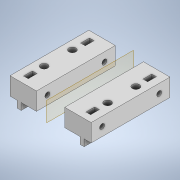
# Autodesk Inventor part: kątnik_v2
Saved by Autodesk Inventor 2022.3 (Build 263350000, 350)
## iProperties
Created: 2022-07-31
Part Number: kątnik_v2
Material: Generic
Document SubType Name: Modeling
Designer: komputer
Density: 1 g/cm^3
Appearance: Default
Author: komputer
Autodesk Inventor part; units mm, degrees
ref_plane "YZ Plane" through (0, 0, 0) normal (1, 0, 0) x (0, 1, 0)
ref_plane "XZ Plane" through (0, 0, 0) normal (0, 1, 0) x (-1, 0, 0)
ref_plane "XY Plane" through (0, 0, 0) normal (0, 0, 1) x (1, 0, 0)
sketch "Sketch1" plane through (0, 0, 0) normal (0, 0, 1) x (1, 0, 0)
  line L0 (1.5, 3.5) -> (1.5, -11.5)
  line L1 (14.5, -11.5) -> (1.5, -11.5)
  line L2 (14.5, -17.3) -> (14.5, -11.5)
  line L3 (18, -17.3) -> (14.5, -17.3)
  line L4 (18, -11.5) -> (18, -17.3)
  line L5 (24, -11.5) -> (18, -11.5)
  line L6 (24, 3.5) -> (24, -11.5)
  line L7 (1.5, 3.5) -> (24, 3.5)
  point P0 (0, 0)
  point P1 (0, 0)
  constraints: 16 end point
extrude "Extrusion1" add sketch "Sketch1" along normal blind 100
sketch "Sketch2" plane through (1.5, -11.5, 0) normal (0, -1, 0) x (1, 0, 0)
  line L0 (0, 0) -> (13, 0) projected
  line L1 (13, 0) -> (13, 100) projected
  line L2 (0, 100) -> (13, 100) projected
  line L3 (0, 0) -> (0, 100) projected
  line L4 (16.5, 0) -> (22.5, 0) projected
  line L5 (22.5, 0) -> (22.5, 100) projected
  line L6 (16.5, 100) -> (22.5, 100) projected
  line L7 (16.5, 0) -> (16.5, 100) projected
  line L8 (22.5, 61) -> (22.5, 0)
  line L9 (22.5, 61) -> (16.5, 61)
  line L10 (16.5, 61) -> (16.5, 56)
  line L11 (16.5, 56) -> (13, 56)
  line L12 (13, 61) -> (13, 56)
  line L13 (13, 61) -> (0, 61)
  line L14 (0, 61) -> (0, 0)
  line L15 (0, 0) -> (13, 0)
  line L16 (13, 0) -> (13, 5)
  line L17 (13, 5) -> (16.5, 5)
  line L18 (16.5, 5) -> (16.5, 0)
  line L19 (16.5, 0) -> (22.5, 0)
  circle A0 centre (15, 13.5) radius 3
  circle A1 centre (15, 47.5) radius 3
  line L20 (16.5, 40.5) -> (16.5, 20.5)
  line L21 (16.5, 20.5) -> (13, 20.5)
  line L22 (13, 40.5) -> (13, 20.5)
  line L23 (13, 40.5) -> (16.5, 40.5)
  line L24 (22.5, 61) -> (22.5, 0)
  line L25 (22.5, 61) -> (16.5, 61)
  line L26 (16.5, 61) -> (16.5, 56)
  line L27 (16.5, 56) -> (13, 56)
  line L28 (13, 61) -> (13, 56)
  line L29 (13, 61) -> (0, 61)
  line L30 (0, 61) -> (0, 0)
  line L31 (0, 0) -> (13, 0)
  line L32 (13, 0) -> (13, 5)
  line L33 (13, 5) -> (16.5, 5)
  line L34 (16.5, 5) -> (16.5, 0)
  line L35 (16.5, 0) -> (22.5, 0)
  circle A2 centre (15, 13.5) radius 3
  circle A3 centre (15, 47.5) radius 3
  line L36 (16.5, 40.5) -> (16.5, 20.5)
  line L37 (16.5, 20.5) -> (13, 20.5)
  line L38 (13, 40.5) -> (13, 20.5)
  line L39 (13, 40.5) -> (16.5, 40.5)
  line L40 (16.5, 20.5) -> (16.5, 30.5)
  line L41 (16.5, 0) -> (16.5, 100) projected
  line L42 (16.5, 30.5) -> (13, 30.5)
  line L43 (13, 0) -> (13, 100) projected
  line L44 (13, 20.5) -> (16.5, 20.5)
  line L45 (15, 30.5) -> (15, 37.5)
  circle A4 centre (15, 37.5) radius 3
  line L46 (15, 37.5) -> (15, 46)
  line L47 (13, 46) -> (16.5, 46)
  line L48 (16.5, 46) -> (16.5, 37.5)
  line L49 (16.5, 37.5) -> (13, 37.5)
  line L50 (13, 37.5) -> (13, 46)
  line L51 (13, 46) -> (16.5, 46)
  line L52 (16.5, 46) -> (16.5, 37.5)
  line L53 (16.5, 37.5) -> (13, 37.5)
  line L54 (13, 37.5) -> (13, 46)
  line L55 (16.5, 5) -> (13, 5)
  line L56 (13, 5) -> (13, 13.5)
  line L57 (13, 13.5) -> (16.5, 13.5)
  line L58 (16.5, 13.5) -> (16.5, 5)
  line L59 (16.5, 13.5) -> (13, 13.5)
  line L60 (13, 13.5) -> (13, 20.5)
  line L61 (13, 20.5) -> (16.5, 20.5)
  line L62 (16.5, 20.5) -> (16.5, 13.5)
  line L63 (13, 30.5) -> (16.5, 30.5)
  line L64 (16.5, 30.5) -> (16.5, 37.5)
  line L65 (16.5, 37.5) -> (13, 37.5)
  line L66 (13, 37.5) -> (13, 30.5)
  line L67 (13, 37.5) -> (16.5, 37.5)
  line L68 (16.5, 37.5) -> (16.5, 46)
  line L69 (16.5, 46) -> (13, 46)
  line L70 (13, 46) -> (13, 37.5)
  line L71 (0, 0) -> (0, 100) projected
  line L72 (22.5, 0) -> (22.5, 100) projected
  line L73 (0, 46) -> (22.5, 46)
  line L74 (22.5, 46) -> (22.5, 100)
  line L75 (22.5, 100) -> (0, 100)
  line L76 (0, 100) -> (0, 46)
  line L77 (16.5, 46) -> (13, 46)
  line L78 (13, 46) -> (13, 30.5)
  line L79 (13, 30.5) -> (16.5, 30.5)
  line L80 (16.5, 30.5) -> (16.5, 46)
  line L81 (13, 46) -> (16.5, 46)
  line L82 (16.5, 46) -> (16.5, 51)
  line L83 (16.5, 51) -> (13, 51)
  line L84 (13, 51) -> (13, 46)
  line L85 (22.5, 51) -> (0, 51)
  point P0 (-1.5, 0)
  point P1 (-9, 27)
  point P2 (16.5, 34.9019)
  point P3 (16.5, 40.0981)
  point P4 (16.5, 46)
  point P5 (13, 46)
  point P6 (0, 51)
  point P7 (13, 51)
  point P8 (13, 100)
  point P9 (13, 100)
  point P10 (13, 51)
  point P11 (13, 51)
  point P12 (12.4019, 46)
  point P13 (13, 49.7361)
  dimension "d2" = 10
  dimension "d4" = 7
  dimension "d5" = 8.5
  dimension "d6" = 5
  constraints: 148 end point, 19 equal length, 11 perpendicular, 9 horizontal, 7 point on line, 5 centre point, 1 coincident, 1 vertical, 8 other
  measures "d2" distance of L36.end L40.end
  measures "d4" distance of L45.start L45.end
  measures "d5" distance of L46.start L46.end
  measures "d6" distance of L82.end L81.end
extrude "Extrusion2" cut sketch "Sketch2" along normal blind 100 contours L1 A0 L7 L17 | L1 L57 L7 A0 | A1 L46 L23 L1 | L1 L47 L46 A1 | L1 A0 L7 L57 | L1 L21 L7 A0 | L23 A4 L1 | L46 L47 L7 A1 | A1 L7 L23 L46 | A4 L46 L49 L1 | L23 L7 A4 | A4 L7 L49 L46 | L1 A4 L45 L42 | L49 L45 A4 L1 | A4 L7 | L49 L7 A4 L45 | L45 A4 L7 L42
extrude "Extrusion3" cut sketch "Sketch2" against normal blind 100 contours L3 L13 L1 L85 | A0 L1 | L1 L57 L7 A0 | L3 L2 L1 L13 | L1 L11 L7 L83 | L1 A0 L7 L57 | L7 A0 | L1 L75 L7 L11 | L7 L9 L5 L85 | A4 L46 L49 L1 | L1 A4 | A4 L7 L49 L46 | L6 L5 L9 L7 | L49 L45 A4 L1 | A4 L7 | L49 L7 A4 L45
extrude "Extrusion4" cut sketch "Sketch2" along normal blind 100 contours L1 L11 L7 L83 | L1 L75 L7 L11
sketch "Sketch4" plane through (0, 0, 0) normal (0, 0, -1) x (-1, 0, 0)
  point P0 (0, 0)
sketch "Sketch5" plane through (0, 0, 0) normal (0, 0, -1) x (-1, 0, 0)
  line L0 (-1.5, 3.5) -> (-1.5, -11.5) projected
  line L1 (-24, 3.5) -> (-1.5, 3.5) projected
  line L2 (-24, -11.5) -> (-24, 3.5) projected
  line L3 (-18, -11.5) -> (-24, -11.5) projected
  line L4 (-18, -17.3) -> (-18, -11.5) projected
  line L5 (-14.5, -17.3) -> (-18, -17.3) projected
  line L6 (-14.5, -11.5) -> (-14.5, -17.3) projected
  line L7 (-1.5, -11.5) -> (-14.5, -11.5) projected
  point P0 (0, 0)
extrude "Extrusion6" add sketch "Sketch5" along normal blind 20
sketch "Sketch6" plane through (1.5, -11.5, 51) normal (0, 0, 1) x (1, 0, 0)
  line L0 (0, 15) -> (22.5, 15) projected
  line L1 (0, 0) -> (0, 15) projected
  line L2 (13, 0) -> (0, 0) projected
  line L3 (13, -5.8) -> (13, 0) projected
  line L4 (16.5, -5.8) -> (13, -5.8) projected
  line L5 (16.5, 0) -> (16.5, -5.8) projected
  line L6 (22.5, 0) -> (16.5, 0) projected
  line L7 (22.5, 15) -> (22.5, 0) projected
  point P0 (-1.5, 11.5)
extrude "Extrusion7" add sketch "Sketch6" along normal blind 20
sketch "Sketch7" plane through (1.5, -11.5, -20) normal (-1, 0, 0) x (0, 0, 1)
  line L0 (91, 15) -> (0, 15) projected
  line L1 (0, 0) -> (0, 15) projected
  line L2 (0, 0) -> (91, 0) projected
  line L3 (91, 15) -> (91, 0) projected
  circle A0 centre (69.75, 7.5) radius 2.1
  line L4 (66, 5.3349) -> (69.75, 3.1699)
  line L5 (69.75, 3.1699) -> (73.5, 5.3349)
  line L6 (73.5, 15) -> (73.5, 5.3349)
  line L7 (66, 15) -> (66, 5.3349)
  line L8 (66, 0) -> (91, 0) projected
  line L9 (66, 0) -> (66, -5.8) projected
  line L10 (66, -5.8) -> (91, -5.8) projected
  line L11 (91, 0) -> (91, -5.8) projected
  line L12 (25, -5.8) -> (25, 0) projected
  line L13 (0, 0) -> (25, 0) projected
  line L14 (0, -5.8) -> (0, 0) projected
  line L15 (0, -5.8) -> (25, -5.8) projected
  line L16 (91, 15) -> (0, 15) projected
  circle A1 centre (21.25, 7.5) radius 2.1
  line L17 (17.5, 5.3349) -> (21.25, 3.1699)
  line L18 (21.25, 3.1699) -> (25, 5.3349)
  line L19 (25, 15) -> (25, 5.3349)
  line L20 (17.5, 15) -> (17.5, 5.3349)
  line L21 (21.25, 3.1699) -> (17.5, 5.3349)
  line L22 (17.5, 5.3349) -> (17.5, 9.6651)
  line L23 (17.5, 9.6651) -> (21.25, 11.8301)
  line L24 (21.25, 11.8301) -> (25, 9.6651)
  line L25 (25, 9.6651) -> (25, 5.3349)
  line L26 (25, 5.3349) -> (21.25, 3.1699)
  line L27 (69.75, 3.1699) -> (66, 5.3349)
  line L28 (66, 5.3349) -> (66, 9.6651)
  line L29 (66, 9.6651) -> (69.75, 11.8301)
  line L30 (69.75, 11.8301) -> (73.5, 9.6651)
  line L31 (73.5, 9.6651) -> (73.5, 5.3349)
  line L32 (73.5, 5.3349) -> (69.75, 3.1699)
  point P0 (20, 11.5)
  constraints: 40 end point, 2 centre point, 2 coincident, 2 point on line, 26 other
extrude "Extrusion9" cut sketch "Sketch7" against normal blind 16.5 contours L6 L5 L4 L7 L29 L30 | L19 L18 L17 L20 L23 L24 | A0 | A1
extrude "Extrusion10" cut sketch "Sketch7" against normal through all contours A0 | A1
extrude "Extrusion11" add sketch "Sketch7" against normal blind 12.5 contours L6 L5 L4 L7 L29 L30 | L19 L18 L17 L20 L23 L24
sketch "Sketch8" plane through (1.5, 3.5, -20) normal (0, 1, 0) x (1, 0, 0)
  line L0 (12.5, -69.75) -> (16.5, -69.75) projected
  line L1 (12.5, -66) -> (16.5, -66) projected
  line L2 (12.5, -73.5) -> (16.5, -73.5) projected
  line L3 (16.5, -67.65) -> (22.5, -67.65) projected
  line L4 (16.5, -71.85) -> (22.5, -71.85) projected
  line L5 (12.5, -73.5) -> (12.5, -69.75) projected
  line L6 (12.5, -69.75) -> (12.5, -66) projected
  line L7 (16.5, -69.75) -> (16.5, -73.5) projected
  line L8 (16.5, -66) -> (16.5, -69.75) projected
  line L9 (12.5, -71.85) -> (0, -71.85) projected
  line L10 (12.5, -67.65) -> (0, -67.65) projected
  line L11 (16.5, -17.5) -> (16.5, -21.25) projected
  line L12 (12.5, -17.5) -> (16.5, -17.5) projected
  line L13 (12.5, -21.25) -> (16.5, -21.25) projected
  line L14 (12.5, -21.25) -> (12.5, -17.5) projected
  line L15 (12.5, -25) -> (12.5, -21.25) projected
  line L16 (16.5, -21.25) -> (16.5, -25) projected
  line L17 (12.5, -25) -> (16.5, -25) projected
  line L18 (16.5, -23.35) -> (22.5, -23.35) projected
  line L19 (16.5, -19.15) -> (22.5, -19.15) projected
  line L20 (12.5, -23.35) -> (0, -23.35) projected
  line L21 (12.5, -19.15) -> (0, -19.15) projected
  point P0 (-1.5, -20)
  dimension "d27" = 6
  measures "d27" distance of L4.start L4.end
extrude "Extrusion12" cut sketch "Sketch8" against normal blind 6
sketch "Sketch9" plane through (1.5, 3.5, -20) normal (0, 1, 0) x (1, 0, 0)
  line L0 (16.5, -17.5) -> (16.5, -25) projected
  line L1 (16.5, -25) -> (12.5, -25) projected
  line L2 (12.5, -25) -> (12.5, -17.5) projected
  line L3 (12.5, -17.5) -> (16.5, -17.5) projected
  line L4 (16.5, -66) -> (16.5, -73.5) projected
  line L5 (16.5, -73.5) -> (12.5, -73.5) projected
  line L6 (12.5, -73.5) -> (12.5, -66) projected
  line L7 (12.5, -66) -> (16.5, -66) projected
  line L8 (22.5, 0) -> (22.5, -91) projected
  line L9 (0, 0) -> (22.5, 0) projected
  line L10 (0, -91) -> (0, 0) projected
  line L11 (22.5, -91) -> (0, -91) projected
  circle A0 centre (15, -57.5) radius 3 projected
  circle A1 centre (15, -33.5) radius 3 projected
  line L12 (12.5, -73.5) -> (16.5, -73.5) projected
  line L13 (14.5, -73.5) -> (14.5, -79)
  line L14 (14.5, -17.5) -> (14.5, -12)
  line L15 (22.5, -91) -> (0, -91) projected
  line L16 (22.5, 0) -> (22.5, -91) projected
  line L17 (0, -91) -> (22.5, -91)
  line L18 (22.5, -91) -> (22.5, -79)
  line L19 (22.5, -79) -> (0, -79)
  line L20 (0, -79) -> (0, -91)
  line L21 (0, 0) -> (22.5, 0) projected
  line L22 (22.5, -12) -> (0, -12)
  line L23 (0, -12) -> (0, 0)
  line L24 (0, 0) -> (22.5, 0)
  line L25 (22.5, 0) -> (22.5, -12)
  point P0 (-1.5, -20)
  dimension "d30" = 5.5
  dimension "d31" = 5.5
  constraints: 20 end point, 4 parallel, 2 horizontal, 2 midpoint, 2 perpendicular, 2 point on line, 2 vertical
  measures "d30" distance of L13.start L13.end
  measures "d31" distance of L14.start L14.end
extrude "Extrusion13" cut sketch "Sketch9" against normal through all contours L8 L22 L10 L9 | L8 L11 L10 L19
sketch "Sketch10" plane through (1.5, -11.5, -8) normal (-1, 0, 0) x (0, 0, 1)
  point P0 (8, 11.5)
sketch "Sketch11" plane through (1.5, -11.5, -8) normal (-1, 0, 0) x (0, 0, 1)
  line L0 (0, 15) -> (0, 0) projected
  line L1 (0, 0) -> (67, 0) projected
  line L2 (67, 0) -> (67, 15) projected
  line L3 (67, 15) -> (0, 15) projected
  circle A0 centre (9.25, 7.5) radius 2.1 projected
  circle A1 centre (57.75, 7.5) radius 2.1 projected
  line L4 (28.5, 0) -> (38.5, 0) projected
  line L5 (33.5, 0) -> (33.5, 15)
  line L6 (67, 15) -> (0, 15) projected
  line L7 (33.5, 7.5) -> (9.25, 7.5)
  line L8 (33.5, 7.5) -> (57.75, 7.5)
  line L9 (67, 0) -> (67, 7.5)
  line L10 (67, 15) -> (67, 0) projected
  point P0 (8, 11.5)
  dimension "d34" = 4.2
  dimension "d35" = 24.25
  dimension "d36" = 15
  constraints: 8 end point, 4 midpoint, 2 horizontal
  measures "d34" diameter of A1
  measures "d35" distance of L7.start L8.end
  measures "d36" distance of L1.end L2.end
sketch "Sketch13" plane through (1.5, 3.5, 59) normal (0, 0, 1) x (1, 0, 0)
  line L0 (0, -15) -> (0, -7)
  line L1 (0, -15) -> (0, 0) projected
  line L2 (0, 0) -> (7, 0)
  line L3 (0, 0) -> (22.5, 0) projected
  line L4 (7, 0) -> (0, -7)
  line L5 (0, 0) -> (7, 0)
  point P0 (-1.5, -3.5)
  dimension "d40" = 8
  dimension "d41" = 7
  constraints: 8 end point, 2 point on line
  measures "d40" distance of L0.start L0.end
  measures "d41" distance of L1.end L2.end
extrude "Extrusion15" cut sketch "Sketch13" against normal through all
sketch "Sketch14" plane through (14.5, -11.5, 5) normal (0, -1, 0) x (1, 0, 0)
  point P0 (-14.5, -5)
extrude "Extrusion16" add sketch "Sketch11" against normal blind 7
sketch "Sketch15" plane through (1.5, -11.5, 59) normal (-1, 0, 0) x (0, 0, 1)
  circle A0 centre (-57.75, 7.5) radius 2.1 projected
  line L0 (-67, 15) -> (-67, 0) projected
  line L1 (-67, 0) -> (0, 0) projected
  line L2 (0, 0) -> (0, 15) projected
  line L3 (0, 15) -> (-67, 15) projected
  circle A1 centre (-9.25, 7.5) radius 2.1 projected
  line L4 (-32.5245, 11.5) -> (-38.3773, 11.5)
  line L5 (-38.3773, 11.5) -> (-38.3773, 6.5245)
  line L6 (-38.3773, 6.5245) -> (-32.5245, 6.5245)
  line L7 (-32.5245, 6.5245) -> (-32.5245, 11.5)
  point P0 (-59, 11.5)
  dimension "d46" = 48.5
  dimension "d47" = 7.5
  constraints: 8 end point, 2 parallel, 1 horizontal, 1 perpendicular
  measures "d46" distance of A0.centre A1.centre
  measures "d47" distance from line of L1 A0.centre
extrude "Extrusion17" add sketch "Sketch15" along normal blind 15 contours L7 L6 L5 L4
mirror "Mirror1" about plane through (-13.5, -2.4877, 23.5491) normal (-1, 0, 0) of "Extrusion1", "Extrusion17", "Extrusion16", "Extrusion15", "Extrusion13", "Extrusion12", "Extrusion11", "Extrusion10", "Extrusion9", "Extrusion7", "Extrusion6", "Extrusion4", "Extrusion3", "Extrusion2"
sketch "Sketch16" plane through (1.5, -4.9755, 26.4755) normal (0, 0, 1) x (1, 0, 0)
  line L0 (0, 4.9755) -> (0, 0) projected
  line L1 (0, 4.9755) -> (-30, 4.9755) projected
  line L2 (-30, 4.9755) -> (-30, 0) projected
  line L3 (0, 0) -> (-30, 0) projected
  point P0 (-1.5, 4.9755)
extrude "Extrusion18" cut sketch "Sketch16" against normal blind 15
sketch "Sketch17" plane through (-28.5, 3.5, 59) normal (0, 1, 0) x (1, 0, 0)
  line L0 (57.9415, 71.5651) -> (20.1329, 71.5651)
  line L1 (20.1329, 71.5651) -> (20.1329, -18.8249)
  line L2 (20.1329, -18.8249) -> (57.9415, -18.8249)
  line L3 (57.9415, -18.8249) -> (57.9415, 71.5651)
  point P0 (28.5, 59)
  constraints: 8 end point, 2 parallel, 1 horizontal, 1 perpendicular
extrude "Extrusion19" cut sketch "Sketch17" against normal through all
ref_plane "Work Plane1" through (-16.5, -11.5, -8) normal (1, 0, 0) x (0, 0, -1)
mirror "Mirror2" about plane through (-16.5, -11.5, -8) normal (1, 0, 0)
body "Solid1"
